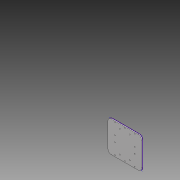
# Autodesk Inventor part: J1_Base
Saved by Autodesk Inventor 2020 (Build 240168000, 168)
## iProperties
Created: 2021-03-23
Part Number: J1_Base
Material: Generic
Document SubType Name: Modeling
Designer: DDeGo
Density: 1 g/cm^3
Appearance: Default
Author: DDeGo
Autodesk Inventor part; units mm, degrees
ref_plane "YZ Plane" through (0, 0, 0) normal (1, 0, 0) x (0, 1, 0)
ref_plane "XZ Plane" through (0, 0, 0) normal (0, 1, 0) x (-1, 0, 0)
ref_plane "XY Plane" through (0, 0, 0) normal (0, 0, 1) x (1, 0, 0)
sketch "Block1" plane through (0, 0, 0) normal (0, 0, 1) x (1, 0, 0)
  circle A0 centre (112.1187, 97.7562) radius 2.75
  line L0 (90.8687, 90.2562) -> (90.8687, 49.9679) construction
  circle A1 centre (83.3687, 50.2562) radius 2.75
  line L1 (75.8687, 49.9679) -> (75.8687, 122.7562) construction
  line L2 (75.8687, 49.9679) -> (90.8687, 49.9679) construction
  circle A2 centre (83.3687, 115.2562) radius 2.75
  line L3 (90.8687, 90.2562) -> (190.8687, 90.2562) construction
  line L4 (75.8687, 122.7562) -> (205.8687, 122.7562) construction
  circle A3 centre (140.8687, 115.2562) radius 2.75
  circle A4 centre (169.6187, 97.7562) radius 2.75
  circle A5 centre (198.3687, 115.2562) radius 2.75
  line L5 (190.8687, 90.2562) -> (190.8687, 40.2562) construction
  line L6 (205.8687, 40.2562) -> (205.8687, 122.7562) construction
  circle A6 centre (198.3687, 50.2562) radius 2.75
  line L7 (205.8687, 40.2562) -> (190.8687, 40.2562) construction
  line L8 (83.3687, 115.2562) -> (140.8687, 115.2562) construction
  line L9 (140.8687, 115.2562) -> (198.3687, 115.2562) construction
  line L10 (198.3687, 115.2562) -> (198.3687, 50.2562) construction
  line L11 (198.3687, 50.2562) -> (83.3687, 50.2562) construction
  line L12 (83.3687, 50.2562) -> (83.3687, 115.2562) construction
  line L13 (112.1187, 115.2562) -> (112.1187, 97.7562) construction
  line L14 (169.6187, 115.2562) -> (169.6187, 97.7562) construction
  line L15 (169.6187, 97.7562) -> (112.1187, 97.7562) construction
  point P0 (142.3997, 87.8737)
  point P1 (140.8687, 90.2562)
  point P2 (140.8687, 90.2562)
  dimension "d9" = 5.5
  dimension "d10" = 57.5
  dimension "d11" = 7.5
  dimension "d12" = 7.5
  dimension "d13" = 7.5
  dimension "d14" = 17.5
  dimension "d15" = 7.5
  dimension "d16" = 10
  dimension "d17" = 65
  dimension "d18" = 7.5
  dimension "d19" = 7.5
  measures "d9" diameter of A0
  measures "d10" distance of L8.start L8.end
  measures "d11" distance between parallel lines of L6 L10
  measures "d12" distance between parallel lines of L4 L9
  measures "d13" distance between parallel lines of L1 L12
  measures "d14" distance of L13.start L13.end
  measures "d15" distance between parallel lines of L3 L15
  measures "d16" distance between parallel lines of L7 L11
  measures "d17" distance of L9.end L10.end
  measures "d18" distance from line of L5 L10.end
  measures "d19" distance between parallel lines of L12 L0
sketch "Sketch1" plane through (0, 0, 0) normal (0, 0, 1) x (1, 0, 0)
  line L0 (60, -90) -> (-60, -90)
  line L1 (-80, -70) -> (-80, 70)
  line L2 (-60, 90) -> (60, 90)
  line L3 (80, 70) -> (80, -70)
  line L4 (80, -90) -> (-80, 90) construction
  line L5 (-80, -90) -> (80, 90) construction
  arc A0 (-60, 90) -> (-80, 70) centre (-60, 70) ccw
  arc A1 (80, 70) -> (60, 90) centre (60, 70) ccw
  arc A2 (60, -90) -> (80, -70) centre (60, -70) ccw
  arc A3 (-80, -70) -> (-60, -90) centre (-60, -70) ccw
  point P0 (0, 0)
  dimension "d1" = 160
  dimension "d2" = 180
  dimension "d3" = 20
  constraints: 12 end point, 8 point on circle, 8 point on line, 8 tangent, 4 centre point, 3 equal radius, 2 midpoint, 2 parallel, 1 horizontal, 1 perpendicular
  measures "d1" distance between parallel lines of L3 L1
  measures "d2" distance between parallel lines of L0 L2
  measures "d3" radius of A0
extrude "Extrusion1" add sketch "Sketch1" along normal blind 6
sketch "Sketch2" plane through (0, 0, 6) normal (0, 0, 1) x (1, 0, 0)
  line L0 (0, 0) -> (-80, 0) construction
  line L1 (-80, 70) -> (-80, -70) projected
  line L2 (0, 0) -> (0, 57.5) construction
  line L3 (60, 90) -> (-60, 90) projected
  circle A0 centre (-28.75, 65) radius 2.75
  line L4 (-50, 57.5) -> (-50, 17.2116) construction
  circle A1 centre (-57.5, 17.5) radius 2.75
  line L5 (-65, 17.2116) -> (-65, 90) construction
  line L6 (-65, 17.2116) -> (-50, 17.2116) construction
  circle A2 centre (-57.5, 82.5) radius 2.75
  line L7 (-50, 57.5) -> (50, 57.5) construction
  line L8 (-65, 90) -> (65, 90) construction
  circle A3 centre (0, 82.5) radius 2.75
  circle A4 centre (28.75, 65) radius 2.75
  circle A5 centre (57.5, 82.5) radius 2.75
  line L9 (50, 57.5) -> (50, 7.5) construction
  line L10 (65, 7.5) -> (65, 90) construction
  circle A6 centre (57.5, 17.5) radius 2.75
  line L11 (65, 7.5) -> (50, 7.5) construction
  line L12 (-57.5, 82.5) -> (0, 82.5) construction
  line L13 (0, 82.5) -> (57.5, 82.5) construction
  line L14 (57.5, 82.5) -> (57.5, 17.5) construction
  line L15 (57.5, 17.5) -> (-57.5, 17.5) construction
  line L16 (-57.5, 17.5) -> (-57.5, 82.5) construction
  line L17 (-28.75, 82.5) -> (-28.75, 65) construction
  line L18 (28.75, 82.5) -> (28.75, 65) construction
  line L19 (28.75, 65) -> (-28.75, 65) construction
  circle A7 centre (-28.75, -65) radius 2.75
  line L20 (-50, -57.5) -> (-50, -17.2116) construction
  circle A8 centre (-57.5, -17.5) radius 2.75
  line L21 (-65, -17.2116) -> (-65, -90) construction
  line L22 (-65, -17.2116) -> (-50, -17.2116) construction
  circle A9 centre (-57.5, -82.5) radius 2.75
  line L23 (-50, -57.5) -> (50, -57.5) construction
  line L24 (-65, -90) -> (65, -90) construction
  circle A10 centre (0, -82.5) radius 2.75
  circle A11 centre (28.75, -65) radius 2.75
  circle A12 centre (57.5, -82.5) radius 2.75
  line L25 (50, -57.5) -> (50, -7.5) construction
  line L26 (65, -7.5) -> (65, -90) construction
  circle A13 centre (57.5, -17.5) radius 2.75
  line L27 (65, -7.5) -> (50, -7.5) construction
  line L28 (-57.5, -82.5) -> (0, -82.5) construction
  line L29 (0, -82.5) -> (57.5, -82.5) construction
  line L30 (57.5, -82.5) -> (57.5, -17.5) construction
  line L31 (57.5, -17.5) -> (-57.5, -17.5) construction
  line L32 (-57.5, -17.5) -> (-57.5, -82.5) construction
  line L33 (-28.75, -82.5) -> (-28.75, -65) construction
  line L34 (28.75, -82.5) -> (28.75, -65) construction
  line L35 (28.75, -65) -> (-28.75, -65) construction
  constraints: 4 end point, 2 horizontal, 1 midpoint, 1 vertical, 2 other
extrude "Extrusion2" cut sketch "Sketch2" against normal through all
equation "\"d12\" = d11"
equation "\"d13\" = d11"
equation "\"d15\" = d11"
equation "\"d18\" = d11"
equation "\"d19\" = d11"
body "Solid1"
